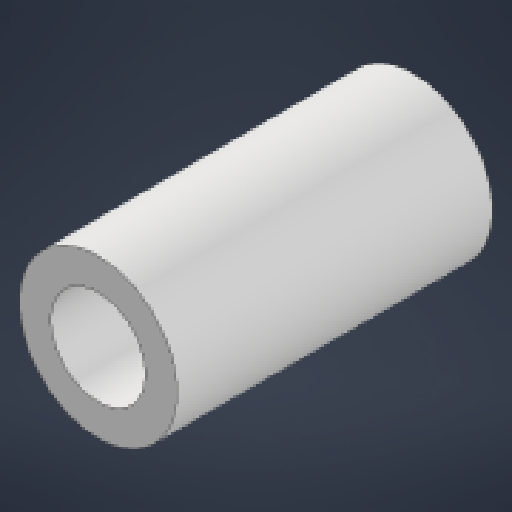
# Autodesk Inventor part: esp_spacer_fixed
Saved by Autodesk Inventor 2024 (Build 280153000, 153)
## iProperties
Created: 2026-03-25
Part Number: esp_spacer_fixed
Material: Generic
Document SubType Name: Modeling
Designer: schar
Density: 1 g/cm^3
Appearance: Default
Author: schar
Autodesk Inventor part; units mm, degrees
ref_plane "YZ Plane" through (0, 0, 0) normal (1, 0, 0) x (0, 1, 0)
ref_plane "XZ Plane" through (0, 0, 0) normal (0, 1, 0) x (-1, 0, 0)
ref_plane "XY Plane" through (0, 0, 0) normal (0, 0, 1) x (1, 0, 0)
sketch "Sketch1" plane through (0, 0, 0) normal (0, 0, 1) x (1, 0, 0)
  circle A0 centre (48.923, 37.7276) radius 1.5 projected
  circle A1 centre (48.923, -37.7276) radius 1.5 projected
  circle A2 centre (83.923, -37.7276) radius 1.5 projected
  circle A3 centre (83.923, 37.7276) radius 1.5 projected
  circle A4 centre (48.923, 37.7276) radius 2.5
  circle A5 centre (83.923, 37.7276) radius 2.5
  circle A6 centre (48.923, -37.7276) radius 2.5
  circle A7 centre (83.923, -37.7276) radius 2.5
  point P0 (0, 0)
  dimension "d0" = 5
  dimension "d1" = 5
  dimension "d2" = 5
  dimension "d3" = 5
  constraints: 4 centre point, 4 coincident
  measures "d0" diameter of A4
  measures "d1" diameter of A5
  measures "d2" diameter of A6
  measures "d3" diameter of A7
extrude "Extrusion1" add sketch "Sketch1" along normal blind 10 contours A4
body "Solid1"
